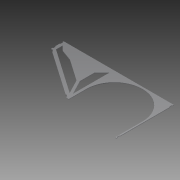
# Autodesk Inventor part: Top
Saved by Autodesk Inventor 2013 (Build 170138000, 138)
## iProperties
Created: 2013-01-27
Part Number: Top
Material: Polycarbonate, Clear
Document SubType Name: Modeling
Designer: Andrew Toennies
Density: 1.2 g/cm^3
Mass: 122.087 g
Surface Area: 749.477 cm^2
Volume: 101.739 cm^3
Author: Andrew Toennies
Autodesk Inventor part; units mm, degrees
ref_plane "YZ Plane" through (0, 0, 0) normal (1, 0, 0) x (0, 1, 0)
ref_plane "XZ Plane" through (0, 0, 0) normal (0, 1, 0) x (-1, 0, 0)
ref_plane "XY Plane" through (0, 0, 0) normal (0, 0, 1) x (1, 0, 0)
sketch "Sketch1" plane through (0, 0, 0) normal (0, 1, 0) x (-1, 0, 0)
  line L0 (0, 0) -> (558.8, 0)
  line L1 (0, 292.1) -> (0, 0)
  arc A0 (6.35, 152.4) -> (292.1, 152.4) centre (149.225, 152.4) ccw
  line L2 (292.1, 152.4) -> (292.1, 241.3)
  line L3 (6.35, 152.4) -> (6.35, 292.1)
  line L4 (0, 292.1) -> (6.35, 292.1)
  line L5 (292.1, 241.3) -> (302.6441, 241.3)
  line L6 (558.8, 0) -> (558.8, 63.5)
  line L7 (558.8, 63.5) -> (302.6441, 241.3)
  point P0 (297.372, 241.3)
  dimension "d0" = 558.8
  dimension "d3" = 285.75
  dimension "d10" = 292.1
  dimension "d14" = 63.5
  dimension "d33" = 241.3
  dimension "d34" = 139.7
  dimension "d37" = 6.35
  constraints: 16 end point, 3 perpendicular, 2 horizontal, 2 parallel, 2 point on circle, 2 tangent, 1 centre point, 1 midpoint, 1 other
  measures "d0" distance of L0.start L0.end
  measures "d3" diameter of A0
  measures "d10" distance between parallel lines of L0 L4
  measures "d14" distance of L0.end L6.end
  measures "d33" distance from line of L0 L5.end
  measures "d34" distance from line of L4 A0.centre
  measures "d37" distance between parallel lines of L1 L3
extrude "Extrusion2" add sketch "Sketch1" along normal blind 3.175
sketch "Sketch2" plane through (-558.8, 0, 0) normal (-1, 0, 0) x (0, 0, 1)
  line L0 (0, 0) -> (63.5, 0) projected
  line L1 (63.5, 0) -> (63.5, 3.175) projected
  line L2 (0, 3.175) -> (63.5, 3.175) projected
  line L3 (0, 0) -> (0, 3.175) projected
  line L4 (6.35, 0) -> (6.35, 3.175)
  line L5 (19.05, 3.175) -> (19.05, 0)
  line L6 (57.15, 3.175) -> (57.15, 0)
  line L7 (44.45, 3.175) -> (44.45, 0)
  dimension "d15" = 6.35
  dimension "d16" = 12.7
  dimension "d17" = 12.7
  dimension "d18" = 6.35
  constraints: 8 end point, 8 point on line, 3 perpendicular, 1 parallel
  measures "d15" distance between parallel lines of L3 L4
  measures "d16" distance between parallel lines of L5 L4
  measures "d17" distance between parallel lines of L6 L7
  measures "d18" distance between parallel lines of L1 L6
extrude "Extrusion3" cut sketch "Sketch2" against normal blind 3.175 contours L4 L2 L5 L0 | L7 L2 L6 L0
sketch "Sketch3" plane through (-558.8, 0, 63.5) normal (-0.5702096, 0, 0.8214993) x (0.8214993, 0, 0.5702096)
  line L0 (0, 0) -> (311.8152, 0) projected
  line L1 (311.8152, 0) -> (311.8152, 3.175) projected
  line L2 (0, 3.175) -> (311.8152, 3.175) projected
  line L3 (0, 0) -> (0, 3.175) projected
  line L4 (6.35, 0) -> (6.35, 3.175)
  line L5 (19.05, 3.175) -> (19.05, 0)
  line L6 (305.4652, 3.175) -> (305.4652, 0)
  line L7 (292.7652, 3.175) -> (292.7652, 0)
  point P0 (422.8455, 0)
  dimension "d21" = 12.7
  dimension "d22" = 6.35
  dimension "d23" = 6.35
  dimension "d24" = 12.7
  constraints: 8 end point, 8 point on line, 4 perpendicular
  measures "d21" distance between parallel lines of L6 L7
  measures "d22" distance between parallel lines of L1 L6
  measures "d23" distance between parallel lines of L4 L3
  measures "d24" distance between parallel lines of L5 L4
extrude "Extrusion4" cut sketch "Sketch3" against normal blind 3.175 contours L4 L2 L5 L0 | L7 L2 L6 L0
sketch "Sketch4" plane through (0, 0, 292.1) normal (1, 0, 0) x (0, 0, -1)
  line L0 (0, 0) -> (292.1, 0) projected
  line L1 (292.1, 0) -> (292.1, 3.175) projected
  line L2 (0, 3.175) -> (292.1, 3.175) projected
  line L3 (285.75, 3.175) -> (285.75, 0)
  line L4 (273.05, 3.175) -> (273.05, 0)
  line L5 (6.35, 3.175) -> (6.35, 0)
  line L6 (19.05, 3.175) -> (19.05, 0)
  dimension "d27" = 12.7
  dimension "d28" = 12.7
  dimension "d29" = 6.35
  dimension "d30" = 254
  constraints: 8 end point, 8 point on line, 3 perpendicular, 1 parallel
  measures "d27" distance between parallel lines of L6 L5
  measures "d28" distance between parallel lines of L4 L3
  measures "d29" distance between parallel lines of L1 L3
  measures "d30" distance between parallel lines of L6 L4
extrude "Extrusion5" cut sketch "Sketch4" against normal blind 3.175 contours L5 L2 L6 L0 | L4 L2 L3 L0
sketch "Sketch6" plane through (0, 3.175, 0) normal (0, 1, 0) x (1, 0, 0)
  line L0 (0, 0) -> (-558.8, 0) projected
  line L1 (-558.8, -19.05) -> (-558.8, -44.45) projected
  line L2 (-543.1504, -74.3625) -> (-318.2936, -230.4375) projected
  line L3 (-307.8606, -237.6792) -> (-302.6441, -241.3) projected
  line L4 (-292.1, -241.3) -> (-292.1, -152.4) projected
  line L5 (-542.925, -55.1945) -> (-316.053, -212.6683)
  line L6 (-304.8, -206.781) -> (-304.8, -21.6803)
  line L7 (-542.925, -55.1945) -> (-542.925, -21.6803)
  line L8 (-533.9447, -12.7) -> (-313.7803, -12.7)
  line L9 (-328.753, -188.3936) -> (-530.225, -48.5502)
  line L10 (-530.225, -48.5502) -> (-530.225, -34.3803)
  line L11 (-521.2447, -25.4) -> (-326.4803, -25.4)
  line L12 (-317.5, -34.3803) -> (-317.5, -182.5063)
  line L13 (-508.6513, -48.0652) -> (-341.453, -164.1189)
  line L14 (-330.2, -158.2316) -> (-330.2, -47.0803)
  line L15 (-339.1803, -38.1) -> (-498.868, -38.1)
  line L16 (-342.9, -59.7803) -> (-342.9, -133.9569)
  line L17 (-354.153, -139.8442) -> (-462.1066, -64.9127)
  line L18 (-463.7816, -50.8) -> (-351.8803, -50.8)
  line L19 (-342.9, -59.7803) -> (-304.8, -21.6803)
  line L20 (-351.8803, -50.8) -> (-313.7803, -12.7)
  line L21 (-463.7816, -50.8) -> (-514.0345, -32.6103)
  line L22 (-462.1066, -64.9127) -> (-521.0155, -43.5897)
  line L23 (-533.9447, -12.7) -> (-514.0345, -32.6103)
  line L24 (-542.925, -21.6803) -> (-521.0155, -43.5897)
  line L25 (-304.8, -206.781) -> (-342.9, -133.9569)
  line L26 (-316.053, -212.6683) -> (-354.153, -139.8442)
  dimension "d38" = 15.875
  dimension "d39" = 12.7
  dimension "d40" = 15.875
  dimension "d41" = 12.7
  dimension "d42" = 12.7
  dimension "d43" = 12.7
  dimension "d44" = 12.7
  dimension "d45" = 12.7
  dimension "d46" = 12.7
  constraints: 44 end point, 12 point on line, 5 perpendicular, 4 parallel, 1 other
  measures "d38" distance between parallel lines of L5 L2
  measures "d39" distance between parallel lines of L4 L6
  measures "d40" distance between parallel lines of L1 L7
  measures "d41" distance between parallel lines of L0 L8
  measures "d42" distance between parallel lines of L8 L11
  measures "d43" distance between parallel lines of L11 L15
  measures "d44" distance between parallel lines of L15 L18
  measures "d45" distance between parallel lines of L14 L16
  measures "d46" distance between parallel lines of L13 L17
extrude "Extrusion6" cut sketch "Sketch6" against normal blind 25.4 contours L7 L24 L10 L9 L26 L5 | L9 L10 L24 L22 L13 L26 | L13 L22 L17 L26 | L25 L12 L19 L6 | L25 L14 L19 L12 | L25 L16 L19 L14
sketch "Sketch7" plane through (0, 3.175, 0) normal (0, 1, 0) x (1, 0, 0)
  line L0 (-342.9, -59.7803) -> (-304.8, -21.6803) projected
  line L1 (-542.925, -21.6803) -> (-521.0155, -43.5897) projected
  line L2 (-521.0155, -43.5897) -> (-462.1066, -64.9127) projected
  line L3 (-307.8606, -237.6792) -> (-302.6441, -241.3) projected
  line L4 (-462.1066, -64.9127) -> (-524.3914, -21.6803)
  line L5 (-524.3914, -21.6803) -> (-542.925, -21.6803)
  line L6 (-342.9, -59.7803) -> (-342.9, -21.6803)
  line L7 (-342.9, -21.6803) -> (-304.8, -21.6803)
  constraints: 8 end point, 2 perpendicular, 1 parallel
extrude "Extrusion7" cut sketch "Sketch7" against normal blind 25.4
sketch "Sketch8" plane through (0, 3.175, 0) normal (0, 1, 0) x (1, 0, 0)
  line L0 (-524.3914, -21.6803) -> (-354.153, -139.8442) projected
  line L1 (-316.053, -212.6683) -> (-542.925, -55.1945) projected
  line L2 (-342.9, -133.9569) -> (-342.9, -21.6803) projected
  line L3 (-355.6, -21.6803) -> (-355.6, -123.3803)
  line L4 (-355.6, -123.3803) -> (-502.1189, -21.6803)
  line L5 (-502.1189, -21.6803) -> (-355.6, -21.6803)
  dimension "d60" = 12.7
  dimension "d61" = 12.7
  constraints: 6 end point, 2 parallel, 1 perpendicular
  measures "d60" distance between parallel lines of L2 L3
  measures "d61" distance between parallel lines of L0 L4
extrude "Extrusion8" cut sketch "Sketch8" against normal blind 25.4
body "Solid2"
